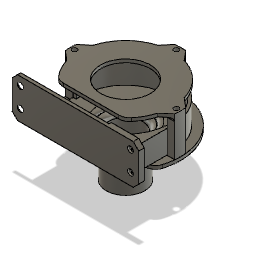
Blower Holder V3 (Model B) (Autodesk Fusion 360 design; units mm, degrees)
Autodesk Fusion 360 part; units mm, degrees
sketch "Sketch1" plane through (0, 0, 0) normal (0, 1, 0) x (1, 0, 0)
  circle A0 centre (0, 0) radius 40
  circle A1 centre (0, 0) radius 20
  circle A2 centre (0, 0) radius 42.5
  dimension "d1" = 80
  dimension "d2" = 40
  dimension "d24" = 85
  constraint coincident A0.centre A1.centre
  constraint concentric A0 A1
  constraint concentric A1 A2
  measures "d1" diameter of A0
  measures "d2" diameter of A1
  measures "d24" diameter of A2
extrude "Extrude1" add sketch "Sketch1" along normal blind 3 contours A0 | A2 makes body 1
sketch "Sketch2" plane through (0, 3, 0) normal (0, 1, 0) x (-1, 0, 0)
  circle A0 centre (0, 0) radius 20
  circle A1 centre (0, 0) radius 42.5
  circle A2 centre (0, 0) radius 40
  circle A3 centre (0, 0) radius 42.5
  dimension "d5" = 80
  dimension "d81" = 2.5
  constraint coincident A0.centre A1.centre
  constraint concentric A1 A2
  measures "d5" diameter of A2
  measures "d81" distance of A1 A2
ref_plane "WorkPlane1" through (0, 21, 0) normal (0, 1, 0) x (-1, 0, 0)
sketch "Sketch3" plane through (0, 21, 0) normal (0, 1, 0) x (1, 0, 0)
  circle A0 centre (0, 0) radius 34
  circle A1 centre (0, 0) radius 37
  dimension "d7" = 68
  dimension "d8" = 74
  constraint coincident A0.centre A1.centre
  measures "d7" diameter of A0
  measures "d8" diameter of A1
extrude "Extrude7" add sketch "Sketch2" along normal up to surface (18 mm away) contours A1 A3 bodies 1
sketch "Sketch9" plane through (0, 0, 0) normal (0, -1, 0) x (1, 0, 0)
  circle A0 centre (0, 0) radius 20
  circle A1 centre (0, 0) radius 42.5
  line L0 (59.9639, 0) -> (-88.3685, 0) construction
  line L1 (0, 0) -> (0, 71.4986) construction
  line L2 (42.5, 0) -> (-42.5, 0)
  line L3 (-42.5, 0) -> (-42.5, 42.5)
  line L4 (-42.5, 42.5) -> (42.5, 42.5)
  line L5 (42.5, 42.5) -> (42.5, 0)
  line L6 (42.5, 0) -> (-42.5, 42.5) construction
  line L7 (-42.5, 0) -> (42.5, 42.5) construction
  point P0 (0, 21.25)
  constraint horizontal L0
  constraint coincident A0.centre L0
  constraint coincident A0.centre A1.centre
  constraint perpendicular L0 L1
  constraint horizontal L2
  constraint perpendicular L2 L3
  constraint parallel L2 L4
  constraint parallel L3 L5
  constraint coincident L0 L2.start
  constraint coincident L6 P0
  constraint coincident L7 P0
  constraint coincident L1 P0
  constraint tangent A1 L5
  constraint tangent A1 L4
extrude "Extrude8" add sketch "Sketch9" against normal up to surface (21 mm away) contours A1 L4 L5 | A1 L3 L4 bodies 1
sketch "Sketch10" plane through (0, 0, 42.5) normal (0, 0, 1) x (1, 0, 0)
  line L0 (42.5, 21) -> (-42.5, 21)
  line L1 (-42.5, 21) -> (-42.5, 0)
  line L2 (-42.5, 0) -> (42.5, 0)
  line L3 (42.5, 0) -> (42.5, 21)
extrude "Extrude9" add sketch "Sketch10" along normal blind 3 bodies 1
sketch "Sketch12" plane through (0, 21, 0) normal (0, 1, 0) x (-1, 0, 0)
  arc A0 (-42.5, 0) -> (42.5, 0) centre (0, 0) ccw
  line L0 (42.5, 0) -> (42.5, 45.5)
  line L1 (-42.5, 45.5) -> (-42.5, 0)
  line L2 (42.5, 0) -> (0.5, 0) construction
  line L3 (0.5, 0) -> (0.5, 45.5)
  line L4 (0.5, 45.5) -> (42.5, 45.5)
  line L5 (42.5, 45.5) -> (42.5, 0)
  line L6 (42.5, 45.5) -> (-42.5, 45.5)
  line L7 (42.5, 5) -> (0.5, 5)
  circle A1 centre (0, 0) radius 40
  dimension "d52" = 5
  dimension "d82" = 42
  constraint horizontal L2
  constraint vertical L3
  constraint horizontal L4
  constraint vertical L5
  constraint coincident A0.end L0.start
  constraint collinear L4 L6
  constraint coincident L0 L7.start
  constraint coincident L3 L7.end
  constraint perpendicular L3 L7
  measures "d52" distance of L2 L7
  measures "d82" distance of L3 L5
extrude "Extrude11" cut sketch "Sketch12" against normal up to surface (18 mm away) contours L0 L3 L4 L5 L6 L7 A1 | L3 L7 A1 picked at (26.2506, 6.8721) bodies 1
ref_plane "WorkPlane2" through (0, 36, 1.5) normal (0, 1, 0) x (0, 0, 1)
sketch "Sketch14" plane through (0, 36, 1.5) normal (0, 1, 0) x (1, 0, 0)
  circle A0 centre (0, 1.5) radius 20
  circle A1 centre (0, 1.5) radius 22.5
  circle A2 centre (0, 1.5) radius 43
  line L0 (-29.5318, -29.7549) -> (29.5318, -29.7549)
  dimension "d45" = 45
  dimension "d46" = 86
  constraint concentric A0 A1
  constraint concentric A0 A2
  constraint coincident A2 L0.start
  constraint coincident A2 L0.end
  constraint horizontal L0
  measures "d45" diameter of A1
  measures "d46" diameter of A2
extrude "Extrude13" add sketch "Sketch14" against normal blind 3 separate body contours A2 L0 picked at (-0.5605, -26.8156) makes body 2
sketch "Sketch16" plane through (0, 36, 0) normal (0, 1, 0) x (-1, 0, 0)
  circle A0 centre (0, 0) radius 22.5
  circle A1 centre (0, 0) radius 50
  line L0 (-50, -5) -> (50, -5)
  line L1 (50, -5) -> (50, 5)
  line L2 (50, 5) -> (-50, 5)
  line L3 (-50, 5) -> (-50, -5)
  line L4 (-50, -5) -> (50, 5) construction
  line L5 (50, -5) -> (-50, 5) construction
  line L6 (-5, -50) -> (5, -50)
  line L7 (5, -50) -> (5, 50)
  line L8 (5, 50) -> (-5, 50)
  line L9 (-5, 50) -> (-5, -50)
  line L10 (-5, -50) -> (5, 50) construction
  line L11 (5, -50) -> (-5, 50) construction
  line L12 (29.5318, 31.2549) -> (-29.5318, 31.2549)
  arc A2 (-29.5318, 31.2549) -> (29.5318, 31.2549) centre (0, 0) ccw
  dimension "d47" = 100
  dimension "d48" = 10
  constraint concentric A0 A1
  constraint horizontal L0
  constraint perpendicular L0 L1
  constraint parallel L0 L2
  constraint parallel L1 L3
  constraint coincident L4 A0.centre
  constraint coincident L5 A0.centre
  constraint coincident A0.centre A1.centre
  constraint tangent A1 L3
  constraint horizontal L6
  constraint perpendicular L6 L7
  constraint parallel L6 L8
  constraint parallel L7 L9
  constraint coincident L10 A0.centre
  constraint coincident L11 A0.centre
  constraint equal L3 L6
  constraint tangent A1 L6
  measures "d47" diameter of A1
  measures "d48" distance of L0.start L2.end
extrude "Extrude14" add sketch "Sketch16" against normal up to surface (36 mm away) contours A1 L0 L2 A2 | A1 L7 L9 A2 | A1 L0 L2 A2 bodies 2
chamfer "Chamfer1" distance 7 angle 45 6 edges at (5, 34.5, -42.7083) (-5, 34.5, -42.7083) (-42.7083, 34.5, -5) (-42.7083, 34.5, 5) (42.7083, 34.5, 5) (42.7083, 34.5, -5) on bodies 2
sketch "Sketch17" plane through (0, 0, 45.5) normal (0, 0, 1) x (1, 0, 0)
  line L0 (-0.5, 3) -> (-42.5, 3)
  line L1 (-42.5, 3) -> (-42.5, 0)
  line L2 (-42.5, 0) -> (42.5, 0)
  line L3 (42.5, 0) -> (42.5, 21)
  line L4 (42.5, 21) -> (-0.5, 21)
  line L5 (-0.5, 21) -> (-0.5, 3)
  line L6 (42.5, 21) -> (57.5, 21)
  line L7 (57.5, 21) -> (57.5, 0)
  line L8 (57.5, 0) -> (42.5, 0)
  line L9 (42.5, 0) -> (42.5, 21)
  dimension "d53" = 15
  constraint horizontal L6
  constraint vertical L7
  constraint horizontal L8
  constraint vertical L9
  constraint coincident L3.end L4.start
  constraint collinear L2 L8
  measures "d53" distance of L3.end L6.end
extrude "Extrude15" add sketch "Sketch17" against normal blind 5 contours L3 L6 L7 L8 L9 bodies 1
sketch "Sketch18" plane through (0, 0, 40.5) normal (0, 0, -1) x (-1, 0, 0)
  line L0 (-57.5, 0) -> (-42.5, 0)
  line L1 (-42.5, 0) -> (-42.5, 21)
  line L2 (-42.5, 21) -> (-57.5, 21)
  line L3 (-57.5, 21) -> (-57.5, 0)
  line L4 (-42.5, 21) -> (-57.5, 0) construction
  circle A0 centre (-50, 10.5) radius 2.65
  dimension "d56" = 5.3
  constraint coincident L1.end L2.start
  constraint coincident L0.start L3.end
  constraint midpoint L4 A0.centre
  measures "d56" diameter of A0
extrude "Extrude16" cut sketch "Sketch18" against normal up to surface (5 mm away) contours A0 bodies 1
fillet "Fillet3" radius 3 9 edges at (-5, 33, -46.2083) (5, 33, -46.2083) (46.2083, 33, -5) (-46.2083, 33, -5) (-46.2083, 33, 5) (46.2083, 33, 5) (-43, 33, 0) (0, 33, -43) (43, 33, 0) on bodies 2
sketch "Sketch27" plane through (0, 0, 0) normal (0, -1, 0) x (1, 0, 0)
  arc A0 (-5, -49.7494) -> (5, -49.7494) centre (0, 0) ccw
  line L0 (5, -49.7494) -> (5, -42.7083)
  line L1 (-5, -42.7083) -> (-5, -49.7494)
  arc A1 (-49.7494, 5) -> (-49.7494, -5) centre (0, 0) ccw
  line L2 (-49.7494, -5) -> (-42.7083, -5)
  line L3 (-42.7083, 5) -> (-49.7494, 5)
  arc A2 (49.7494, -5) -> (49.7494, 5) centre (0, 0) ccw
  line L4 (-49.7494, 5) -> (-42.7083, -5) construction
  circle A3 centre (-46.2288, 0) radius 2.25
  line L5 (-5, -42.7083) -> (5, -49.7494) construction
  line L6 (49.7494, 5) -> (42.7083, -5) construction
  circle A4 centre (46.2288, 0) radius 2.25
  circle A5 centre (0, -46.2288) radius 2.25
  line L7 (42.7083, -5) -> (49.7494, -5)
  line L8 (49.7494, 5) -> (42.7083, 5)
  arc A6 (-5, -42.7083) -> (5, -42.7083) centre (0, 0) ccw
  arc A7 (-42.7083, 5) -> (-42.7083, -5) centre (0, 0) ccw
  arc A8 (42.7083, -5) -> (42.7083, 5) centre (0, 0) ccw
  dimension "d84" = 4.5
  constraint coincident A1.start L3.end
  constraint coincident L2.end L4.end
  constraint midpoint L4 A3.centre
  constraint coincident L1.start L5.start
  constraint coincident A0.end L0.start
  constraint coincident A2.end L6.start
  constraint midpoint L6 A4.centre
  constraint midpoint L5 A5.centre
  constraint equal A4 A5
  constraint equal A3 A4
  measures "d84" diameter of A3
extrude "Extrude23" cut sketch "Sketch27" against normal up to surface (36 mm away) contours A3 | A4 | A5 bodies 2
sketch "Sketch19" plane through (0, 0, 45.5) normal (0, 0, 1) x (1, 0, 0)
  line L0 (57.5, 0) -> (57.5, 21)
  line L1 (57.5, 21) -> (-0.5, 21)
  line L2 (-0.5, 21) -> (-0.5, 3)
  line L3 (-0.5, 3) -> (-42.5, 3)
  line L4 (-42.5, 3) -> (-42.5, 0)
  line L5 (-42.5, 0) -> (57.5, 0)
  circle A0 centre (50, 10.5) radius 2.65
  line L6 (57.5, 21) -> (27.5, 21)
  line L7 (27.5, 21) -> (27.5, 36)
  line L8 (27.5, 36) -> (57.5, 36)
  line L9 (57.5, 36) -> (57.5, 21)
  point P0 (42.5, 0)
  point P1 (42.5, 21)
  dimension "d61" = 15
  dimension "d62" = 30
  constraint horizontal L6
  constraint vertical L7
  constraint horizontal L8
  constraint vertical L9
  constraint collinear L0 L9
  constraint collinear L1 L6
  measures "d61" distance of L0.end L8.end
  measures "d62" distance of L7.end L8.end
extrude "Extrude17" add sketch "Sketch19" against normal blind 5 contours L1 L6 L7 L8 L9 bodies 1
sketch "Sketch20" plane through (0, 0, 40.5) normal (0, 0, -1) x (-1, 0, 0)
  circle A0 centre (-50, 10.5) radius 2.65
  line L0 (-57.5, 0) -> (-42.5, 0)
  line L1 (-42.5, 0) -> (-42.5, 21)
  line L2 (-42.5, 21) -> (-27.5, 21)
  line L3 (-27.5, 21) -> (-27.5, 36)
  line L4 (-27.5, 36) -> (-57.5, 36)
  line L5 (-57.5, 36) -> (-57.5, 0)
  line L6 (-42.5, 21) -> (-57.5, 21) construction
  line L7 (-42.5, 21) -> (-57.5, 36) construction
  circle A1 centre (-50, 28.5) radius 2.65
  constraint coincident L1.end L2.start
  constraint coincident L5 L6.end
  constraint perpendicular L5 L6
  constraint coincident L4.end L5.start
  constraint midpoint L7 A1.centre
  constraint equal A0 A1
extrude "Extrude18" cut sketch "Sketch20" against normal up to surface (5 mm away) contours A1 bodies 1
sketch "Sketch22" plane through (0, 0, 45.5) normal (0, 0, 1) x (1, 0, 0)
  circle A0 centre (50, 10.5) radius 2.65
  circle A1 centre (50, 28.5) radius 2.65
  line L0 (-0.5, 21) -> (-0.5, 3)
  line L1 (-0.5, 3) -> (-42.5, 3)
  line L2 (-42.5, 3) -> (-42.5, 0)
  line L3 (-42.5, 0) -> (57.5, 0)
  line L4 (57.5, 0) -> (57.5, 36)
  line L5 (57.5, 36) -> (27.5, 36)
  line L6 (27.5, 21) -> (-0.5, 21)
  line L7 (-57.5, 0) -> (27.5, 0)
  line L8 (27.5, 0) -> (27.5, 36)
  line L9 (27.5, 36) -> (-57.5, 36)
  line L10 (-57.5, 36) -> (-57.5, 0)
  line L11 (27.5, 36) -> (27.5, 21)
  dimension "d73" = 15
  constraint horizontal L7
  constraint vertical L8
  constraint horizontal L9
  constraint vertical L10
  constraint collinear L5 L9
  constraint coincident L5.end L8
  constraint collinear L3 L7
  measures "d73" distance of L2.end L10
extrude "Extrude19" add sketch "Sketch22" against normal blind 3 contours L0 L1 L2 L3 L6 L7 L8 | L0 L1 L2 L6 L7 L8 L9 L10 L11 bodies 1
sketch "Sketch23" plane through (0, 0, 45.5) normal (0, 0, 1) x (1, 0, 0)
  line L0 (57.5, 0) -> (57.5, 36)
  line L1 (57.5, 36) -> (-57.5, 36)
  line L2 (-57.5, 36) -> (-57.5, 0)
  line L3 (-57.5, 0) -> (57.5, 0)
  circle A0 centre (50, 28.5) radius 2.65
  circle A1 centre (50, 10.5) radius 2.65
  line L4 (50, 28.5) -> (-57.5, 28.5) construction
  line L5 (50, 10.5) -> (-57.5, 10.5) construction
  circle A2 centre (-50, 28.5) radius 2.65
  line L6 (-50, 28.5) -> (-50, 10.5) construction
  circle A3 centre (-50, 10.5) radius 2.65
  line L7 (50, 28.5) -> (57.5, 28.5)
  line L8 (-50, 28.5) -> (-57.5, 28.5)
  constraint coincident A0.centre L4.start
  constraint coincident L2 L4.end
  constraint perpendicular L2 L4
  constraint coincident A1.centre L5.start
  constraint coincident L2 L5.end
  constraint perpendicular L2 L5
  constraint coincident L4 A2.centre
  constraint coincident A2.centre L6.start
  constraint coincident L5 L6.end
  constraint perpendicular L5 L6
  constraint coincident L6.end A3.centre
  constraint equal A0 A2
  constraint equal A2 A3
  constraint coincident L0 L7.end
  constraint perpendicular L0 L7
  constraint equal L7 L8
extrude "Extrude20" cut sketch "Sketch23" against normal up to surface (3 mm away) contours A2 | A3 bodies 1
chamfer "Chamfer4" distance 5 angle 45 4 edges at (57.5, 36, 43) (57.5, 0, 43) (-57.5, 0, 44) (-57.5, 36, 44) on bodies 1
chamfer "Chamfer5" distance 3 angle 45 4 edges at (52.4707, 29.4583, 40.5) (52.4707, 11.4583, 40.5) (-52.4707, 27.5417, 42.5) (-52.4707, 9.5417, 42.5) on bodies 1
sketch "Sketch24" plane through (0, 0, 0) normal (0, -1, 0) x (1, 0, 0)
  line L0 (-52.5, 45.5) -> (-52.5, 42.5)
  line L1 (-52.5, 42.5) -> (-42.5, 42.5)
  line L2 (-42.5, 42.5) -> (-42.5, 0)
  arc A0 (-42.5, 0) -> (42.5, 0) centre (0, 0) ccw
  line L3 (42.5, 0) -> (42.5, 40.5)
  line L4 (42.5, 40.5) -> (52.5, 40.5)
  line L5 (52.5, 40.5) -> (52.5, 45.5)
  line L6 (52.5, 45.5) -> (-52.5, 45.5)
  circle A1 centre (0, 0) radius 20
  circle A2 centre (0, 0) radius 17.5
  circle A3 centre (0, 0) radius 50.635
  dimension "d76" = 35
  constraint concentric A0 A2
  constraint concentric A0 A3
  measures "d76" diameter of A2
extrude "Extrude21" add sketch "Sketch24" along normal blind 3 separate body contours L2 A0 L3 L6 A3 | L2 A0 L3 A3 makes body 3
sketch "Sketch28" plane through (0, 0, 0) normal (0, -1, 0) x (1, 0, 0)
  line L0 (-52.5, 45.5) -> (-52.5, 42.5)
  line L1 (-52.5, 42.5) -> (-42.5, 42.5)
  line L2 (-42.5, 42.5) -> (-42.5, 0)
  arc A0 (-42.5, 0) -> (42.5, 0) centre (0, 0) ccw
  line L3 (42.5, 0) -> (42.5, 40.5)
  line L4 (42.5, 40.5) -> (52.5, 40.5)
  line L5 (52.5, 40.5) -> (52.5, 45.5)
  line L6 (52.5, 45.5) -> (-52.5, 45.5)
  circle A1 centre (0, 0) radius 20
  circle A2 centre (0, 0) radius 50
  arc A3 (-5, -49.7494) -> (5, -49.7494) centre (0, 0) ccw
  line L7 (-45.2597, 21.25) -> (45.2597, 21.25)
  point P0 (0.0698, -50)
  constraint concentric A0 A2
  constraint coincident A2 P0
  constraint coincident A3 P0
  constraint coincident A2 L7.start
  constraint coincident A2 L7.end
  constraint perpendicular L3 L7
extrude "Extrude24" add sketch "Sketch28" along normal blind 3 separate body contours L2 A0 L3 L7 | L2 A0 L3 A2 A3 L7 | A1 makes body 4
sketch "Sketch29" plane through (0, -3, 0) normal (0, -1, 0) x (1, 0, 0)
  arc A0 (-45.2597, 21.25) -> (45.2597, 21.25) centre (0, 0) ccw
  line L0 (45.2597, 21.25) -> (-45.2597, 21.25)
  circle A1 centre (0, 0) radius 15.5
  dimension "d89" = 31
  constraint concentric A0 A1
  measures "d89" diameter of A1
extrude "Extrude25" cut sketch "Sketch29" against normal up to surface (3 mm away) contours A1 bodies 4
sketch "Sketch30" plane through (0, -3, 0) normal (0, -1, 0) x (1, 0, 0)
  circle A0 centre (0, 0) radius 15.5
  arc A1 (-45.2597, 21.25) -> (45.2597, 21.25) centre (0, 0) ccw
  line L0 (45.2597, 21.25) -> (-45.2597, 21.25)
  circle A2 centre (0, 0) radius 17.5
  dimension "d92" = 2
  constraint concentric A0 A2
  measures "d92" distance of A0 A2
extrude "Extrude26" add sketch "Sketch30" along normal blind 40 contours A2 bodies 4
fillet "Fillet4" radius 10 1 edges at (-16.3157, -3, 6.3283) on bodies 4
fillet "Fillet5" radius 5 1 edges at (-18.6465, 3, -7.2323) on bodies 1
sketch "Sketch31" plane through (0, -3, 0) normal (0, -1, 0) x (1, 0, 0)
  arc A0 (-17.4553, 21.25) -> (17.4553, 21.25) centre (0, 0) ccw
  line L0 (-17.4553, 21.25) -> (-45.2597, 21.25)
  arc A1 (-45.2597, 21.25) -> (45.2597, 21.25) centre (0, 0) ccw
  line L1 (45.2597, 21.25) -> (17.4553, 21.25)
  circle A2 centre (-46.2288, 0) radius 2.25
  circle A3 centre (0, -46.2288) radius 2.25
  circle A4 centre (46.2288, 0) radius 2.25
extrude "Extrude27" cut sketch "Sketch31" against normal up to surface (3 mm away) contours A2 | A3 | A4 bodies 4
fillet "Fillet6" radius 10 4 edges at (29.5318, 34.5, 31.2549) (-29.5318, 34.5, 31.2549) (45.2597, -1.5, 21.25) (-45.2597, -1.5, 21.25) on bodies 2 4
fillet "Fillet7" radius 5 1 edges at (-14.4511, 0, -5.605) on bodies 4
copy_body "Body->Comp1" bodies 1 removing the originals makes body 5 in component "Body"
copy_body "Body->Comp2" bodies 2 removing the originals makes body 6 in component "Top"
copy_body "Body->Comp3" bodies 3 removing the originals makes body 7 in component "Component"
copy_body "Body->Comp4" bodies 4 removing the originals makes body 8 in component "Bottom"
component "Body" placed x (1, 0, 0) y (0, 1, 0) z (0, 0, 1) at (0, 0, 0)
component "Top" placed x (1, 0, 0) y (0, 1, 0) z (0, 0, 1) at (0, 0, 0)
component "Component" placed x (1, 0, 0) y (0, 1, 0) z (0, 0, 1) at (0, 0, 0)
component "Bottom" placed x (1, 0, 0) y (0, 1, 0) z (0, 0, 1) at (0, 0, 0)
named bodies: "Body", "Top", "Bottom"
